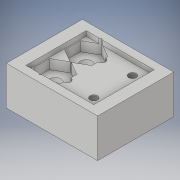
# Autodesk Inventor part: CurrentMonitorBlock
Saved by Autodesk Inventor 2019 (Build 230136000, 136)
## iProperties
Created: 2019-10-11
Part Number: CurrentMonitorBlock
Material: Generic
Document SubType Name: Modeling
Designer: james
Density: 1 g/cm^3
Appearance: Default
Author: james
Autodesk Inventor part; units mm, degrees
ref_plane "YZ Plane" through (0, 0, 0) normal (1, 0, 0) x (0, 1, 0)
ref_plane "XZ Plane" through (0, 0, 0) normal (0, 1, 0) x (-1, 0, 0)
ref_plane "XY Plane" through (0, 0, 0) normal (0, 0, 1) x (1, 0, 0)
sketch "Sketch1" plane through (0, 0, 0) normal (0, 1, 0) x (-1, 0, 0)
  line L0 (8.2338, 13.4805) -> (-21.7662, 13.4805)
  line L1 (-21.7662, 13.4805) -> (-21.7662, -11.5195)
  line L2 (-21.7662, -11.5195) -> (8.2338, -11.5195)
  line L3 (8.2338, -11.5195) -> (8.2338, 13.4805)
  point P0 (0, 0)
  dimension "d0" = 25
  dimension "d1" = 30
  constraints: 8 end point, 2 parallel, 1 horizontal, 1 perpendicular
  measures "d0" distance of L2.end L0.start
  measures "d1" distance of L0.start L0.end
extrude "Extrusion1" add sketch "Sketch1" along normal blind 12.7
sketch "Sketch2" plane through (0, 0, 0) normal (0, -1, 0) x (1, 0, 0)
  line L0 (-8.2338, 13.4805) -> (21.7662, 13.4805) projected
  line L1 (21.7662, 13.4805) -> (21.7662, -11.5195) projected
  point P0 (0, 0)
  point P1 (19.2262, 10.3055)
  point P2 (19.2262, -8.7445)
  point P3 (-6.1738, -8.7445)
  point P4 (-6.1738, 10.3055)
  dimension "d4" = 3.175
  dimension "d5" = 2.54
  dimension "d6" = 19.05
  dimension "d7" = 2.54
  dimension "d8" = 25.4
  dimension "d9" = 3.175
  dimension "d10" = 19.05
  dimension "d11" = 0
  measures "d4" distance from line of L0 point (19.226, 10.306)
  measures "d5" distance from line of L1 point (19.226, 10.306)
  measures "d6" distance of point (19.226, -8.744) point (19.226, 10.306)
  measures "d7" distance from line of L1 point (19.226, -8.744)
  measures "d8" distance of point (-6.174, 10.306) point (19.226, 10.306)
  measures "d9" distance from line of L0 point (-6.174, 10.306)
  measures "d10" distance of point (-6.174, 10.306) point (-6.174, -8.744)
  measures "d11" horizontal distance of point (-6.174, 10.306) point (-6.174, -8.744)
hole "Hole1" at (19.2262, 0, 10.3055) at (19.2262, 0, -8.7445) at (-6.1738, 0, -8.7445) at (-6.1738, 0, 10.3055) direction (0, 1, 0) diameter 2.6416 depth 10 tip angle 118.188 thread size "6-32 UNC" class "2B" standard "ANSI Unified Screw Threads"
sketch "Sketch3" plane through (0, 12.7, 0) normal (0, 1, 0) x (1, 0, 0)
  line L0 (-4.3838, -10.8805) -> (17.9162, -10.8805)
  line L1 (17.9162, -10.8805) -> (17.9162, 8.9195)
  line L2 (17.9162, 8.9195) -> (-4.3838, 8.9195)
  line L3 (-4.3838, 8.9195) -> (-4.3838, -10.8805)
  line L4 (-8.2338, 11.5195) -> (-8.2338, -13.4805) projected
  line L5 (21.7662, 11.5195) -> (-8.2338, 11.5195) projected
  point P0 (0, 0)
  dimension "d19" = 19.8
  dimension "d20" = 22.3
  dimension "d22" = 3.85
  dimension "d23" = 2.6
  constraints: 8 end point, 2 parallel, 1 horizontal, 1 perpendicular
  measures "d19" distance of L2.end L0.start
  measures "d20" distance of L0.start L0.end
  measures "d22" distance between parallel lines of L4 L3
  measures "d23" distance between parallel lines of L5 L2
extrude "Extrusion2" cut sketch "Sketch3" against normal blind 1.57
sketch "Sketch4" plane through (0, 11.13, 0) normal (0, 1, 0) x (1, 0, 0)
  line L0 (-4.3838, -10.8805) -> (-4.3838, 8.9195) projected
  line L1 (17.9162, -10.8805) -> (-4.3838, -10.8805) projected
  line L2 (17.9162, 8.9195) -> (17.9162, -10.8805) projected
  point P0 (0, 0)
  point P1 (14.4162, -7.3805)
  point P2 (14.4162, 5.3195)
  point P3 (4.8762, 4.7295)
  point P4 (4.8762, -6.7005)
  dimension "d28" = 0
  dimension "d30" = 9.26
  dimension "d31" = 4.18
  dimension "d32" = 11.43
  dimension "d33" = 3.5
  dimension "d34" = 3.5
  dimension "d35" = 3.5
  dimension "d36" = 12.7
  measures "d28" horizontal distance of point (4.876, -6.701) point (4.876, 4.729)
  measures "d30" distance from line of point (4.876, -6.701) L0
  measures "d31" distance from line of L1 point (4.876, -6.701)
  measures "d32" distance of point (4.876, 4.729) point (4.876, -6.701)
  measures "d33" distance from line of L1 point (14.416, -7.381)
  measures "d34" distance from line of L2 point (14.416, -7.381)
  measures "d35" distance from line of L2 point (14.416, 5.319)
  measures "d36" distance of point (14.416, -7.381) point (14.416, 5.319)
hole "Hole2" at (14.4162, 11.13, 7.3805) at (14.4162, 11.13, -5.3195) at (4.8762, 11.13, -4.7295) at (4.8762, 11.13, 6.7005) direction (0, -1, 0) diameter 2.4638 depth 6 tip angle 118.188
sketch "Sketch5" plane through (0, 11.13, 0) normal (0, 1, 0) x (1, 0, 0)
  line L0 (17.9162, -10.8805) -> (-4.3838, -10.8805) projected
  line L1 (-4.3838, -10.8805) -> (-4.3838, 8.9195) projected
  line L2 (0.4262, -0.8744) -> (4.9262, -3.4724)
  line L3 (4.9262, -3.4724) -> (4.9262, -8.6686)
  line L4 (4.9262, -8.6686) -> (0.4262, -11.2667)
  line L5 (0.4262, -11.2667) -> (-4.0738, -8.6686)
  line L6 (-4.0738, -8.6686) -> (-4.0738, -3.4724)
  line L7 (-4.0738, -3.4724) -> (0.4262, -0.8744)
  line L8 (0.4262, -1.1067) -> (-4.0738, 1.4914)
  line L9 (-4.0738, 1.4914) -> (-4.0738, 6.6876)
  line L10 (-4.0738, 6.6876) -> (0.4262, 9.2856)
  line L11 (0.4262, 9.2856) -> (4.9262, 6.6876)
  line L12 (4.9262, 6.6876) -> (4.9262, 1.4914)
  line L13 (4.9262, 1.4914) -> (0.4262, -1.1067)
  point P0 (0.4262, -6.0705)
  point P1 (0.4262, 4.0895)
  point P2 (0.4262, -6.0705)
  point P3 (0.4262, 4.0895)
  dimension "d49" = 4.81
  dimension "d50" = 4.81
  dimension "d51" = 10.16
  dimension "d52" = 0
  dimension "d53" = 9
  dimension "d54" = 9
  constraints: 24 end point, 2 coincident, 26 other
  measures "d49" distance from line of L1 point (0.426, -6.071)
  measures "d50" distance from line of L0 point (0.426, -6.071)
  measures "d51" distance of point (0.426, -6.071) point (0.426, 4.089)
  measures "d52" horizontal distance of point (0.426, -6.071) point (0.426, 4.089)
  measures "d53" distance between parallel lines of L3 L6
  measures "d54" distance between parallel lines of L12 L9
extrude "Extrusion3" cut sketch "Sketch5" along normal mid plane 6.35
sketch "Sketch7" plane through (0, 7.955, 0) normal (0, 1, 0) x (1, 0, 0)
  line L0 (0.2251, -0.9905) -> (-4.0738, 1.4914) projected
  line L1 (-4.0738, -3.4724) -> (0.2251, -0.9905) projected
  line L2 (-4.0738, -8.6686) -> (-4.0738, -3.4724) projected
  line L3 (-0.2426, -10.8805) -> (-4.0738, -8.6686) projected
  line L4 (4.9262, -8.6686) -> (1.0951, -10.8805) projected
  line L5 (4.9262, -7.9314) -> (4.9262, -8.6686) projected
  line L6 (4.9262, -3.4724) -> (4.9262, -5.4696) projected
  line L7 (0.6274, -0.9905) -> (4.9262, -3.4724) projected
  line L8 (4.9262, 1.4914) -> (0.6274, -0.9905) projected
  line L9 (4.9262, 3.4986) -> (4.9262, 1.4914) projected
  line L10 (4.9262, 6.6876) -> (4.9262, 5.9604) projected
  line L11 (1.0604, 8.9195) -> (4.9262, 6.6876) projected
  line L12 (-4.0738, 6.6876) -> (-0.208, 8.9195) projected
  line L13 (-4.0738, 1.4914) -> (-4.0738, 6.6876) projected
  circle A0 centre (0.4262, -6.0705) radius 1.8986
  circle A1 centre (0.4262, 4.0895) radius 1.8986
  point P0 (0, 0)
  dimension "d57" = 3.7973
  dimension "d58" = 3.7973
  constraints: 2 centre point
  measures "d57" diameter of A1
  measures "d58" diameter of A0
extrude "Extrusion4" cut sketch "Sketch7" against normal blind 25.4
body "Solid1"
